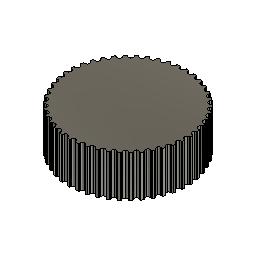
gear_46z (Autodesk Fusion 360 design; units mm, degrees)
Autodesk Fusion 360 part; units mm, degrees
sketch "Sketch1" plane through (0, 0, 0) normal (0, 0, 1) x (1, 0, 0) in component "gt2 pulley"
  circle A0 centre (0, 0) radius 14.6423 construction
  circle A1 centre (0, 0) radius 13.6383 construction
  line L0 (0, 0) -> (0, 14.6423) construction
  line L1 (0, 0) -> (0.9992, 14.6081) construction
  line L2 (0, 0) -> (1.4077, 14.5744) construction
  circle A2 centre (0, 0) radius 14.3883 construction
  arc A3 (0.386, 14.2474) -> (0.4514, 13.9588) centre (1.3833, 14.3216) ccw
  circle A4 centre (0, 0) radius 14.2383 construction
  arc A5 (0.2389, 14.3863) -> (0, 14.3883) centre (0, 0) ccw
  arc A6 (0.386, 14.2474) -> (0.2389, 14.3863) centre (0.2364, 14.2363) ccw
  arc A7 (0.4514, 13.9588) -> (0.9307, 13.6065) centre (0.9686, 14.1602) ccw
  arc A8 (0, 14.3883) -> (-0.2389, 14.3863) centre (0, 0) ccw
  arc A9 (-0.2389, 14.3863) -> (-0.386, 14.2474) centre (-0.2364, 14.2363) ccw
  arc A10 (-0.4514, 13.9588) -> (-0.386, 14.2474) centre (-1.3833, 14.3216) ccw
  arc A11 (-0.9309, 13.6064) -> (-0.4514, 13.9588) centre (-0.9686, 14.1602) ccw
  arc A12 (0.9307, 13.6065) -> (-0.9307, 13.6065) centre (0, 0) ccw
  point P0 (1.3833, 14.3216)
  point P1 (0, 14.3883)
  dimension "d18" = 29.2845
  dimension "d19" = 3.913
  dimension "d22" = 1.004
  dimension "d24" = 0.75
  dimension "d26" = 1
  dimension "d27" = 0.15
  dimension "d28" = 0.15
  dimension "d47" = 0.555
  dimension "d52" = 3.812
  constraint coincident A0.centre A1.centre
  constraint coincident A0 L0.end
  constraint vertical L0
  constraint coincident A0 L1.end
  constraint coincident A0 L2.end
  constraint concentric A1 A2
  constraint coincident A1 A7.end
  constraint coincident L1 A7.end
  constraint coincident A2 P0
  constraint coincident L2 P0
  constraint coincident P0 A3.centre
  constraint coincident A2 P1
  constraint coincident L0 P1
  constraint concentric A2 A4
  constraint coincident P1 A5.end
  constraint coincident A4 A6.centre
  constraint coincident A3.start A6.start
  constraint tangent A3 A6
  constraint tangent A3 A7
  constraint symmetric L0 A7.end A12.end
  constraint symmetric L0 A3.start A9.end
  constraint symmetric L0 A3.end A10.start
  constraint symmetric L0 A3 A10
  constraint symmetric L0 A5.start A8.end
  constraint symmetric L0 P1 A5.end
  constraint symmetric L0 A5 A8
  constraint symmetric L0 A6 A9
  constraint symmetric L0 A7 A11
  constraint coincident A1 A11.start
  constraint tangent A1 A7
  constraint coincident L1 A7.centre
  measures "d18" diameter of A0
  measures "d19" angle of L0 L1
  measures "d22" distance of A0 A1
  measures "d24" distance of A1 A2
  measures "d26" radius of A3
  measures "d27" distance of A2 A4
  measures "d28" radius of A6
  measures "d47" radius of A7
extrude "Extrude1" add sketch "Sketch1" along normal blind 10 makes body 1
pattern_circular "C-Pattern1" count 46 over 360 about axis through (0, 0, 1.75) along (0, 0, 1) of bodies 1 makes body 2 at (-2.572, 13.3935, 6.6667) makes body 3 at (-3.7792, 13.1042, 6.6667) makes body 4 at (-4.7617, 12.78, 3.3333) makes body 5 at (-7.1745, 11.5986, 6.6667) makes body 6 at (-8.0331, 11.0214, 3.3333) makes body 7 at (-9.459, 9.8249, 3.3333) makes body 8 at (-11.544, 7.2621, 6.6667) makes body 9 at (-12.1565, 6.1823, 6.6667) makes body 10 at (-12.5902, 5.243, 3.3333) makes body 11 at (-13.3737, 2.6733, 6.6667) makes body 12 at (-13.5379, 1.6518, 3.3333) makes body 13 at (-13.6367, -0.207, 3.3333) makes body 14 at (-13.1868, -3.48, 6.6667) makes body 15 at (-12.5901, -5.2432, 6.6667) makes body 16 at (-12.4253, -5.6227, 3.3333) makes body 17 at (-11.5439, -7.2623, 3.3333) makes body 18 at (-10.4475, -8.7665, 3.3333) makes body 19 at (-8.033, -11.0215, 6.6667) makes body 20 at (-6.9975, -11.7063, 6.6667) makes body 21 at (-6.09, -12.203, 3.3333) makes body 22 at (-4.3716, -12.9186, 3.3333) makes body 23 at (-2.5718, -13.3936, 3.3333) makes body 24 at (0.1036, -13.6379, 6.6667) makes body 25 at (2.572, -13.3935, 6.6667) makes body 26 at (3.7792, -13.1042, 6.6667) makes body 27 at (4.7617, -12.78, 3.3333) makes body 28 at (7.1745, -11.5986, 6.6667) makes body 29 at (8.0331, -11.0214, 3.3333) makes body 30 at (9.459, -9.8249, 3.3333) makes body 31 at (11.544, -7.2621, 6.6667) makes body 32 at (11.759, -6.9085, 3.3333) makes body 33 at (12.8851, -4.4694, 6.6667) makes body 34 at (13.3737, -2.6733, 6.6667) makes body 35 at (13.5379, -1.6518, 3.3333) makes body 36 at (13.6367, 0.207, 3.3333) makes body 37 at (13.1868, 3.48, 6.6667) makes body 38 at (13.0752, 3.8785, 3.3333) makes body 39 at (12.4253, 5.6227, 3.3333) makes body 40 at (11.5439, 7.2623, 3.3333) makes body 41 at (10.4475, 8.7665, 3.3333) makes body 42 at (8.033, 11.0215, 6.6667) makes body 43 at (7.6949, 11.2601, 3.3333) makes body 44 at (6.09, 12.203, 3.3333) makes body 45 at (4.3716, 12.9186, 3.3333) makes body 46 at (2.5718, 13.3936, 3.3333)
sketch "Sketch2" plane through (0, 0, 10) normal (0, 0, 1) x (-1, 0, 0)
  arc A0 (-10.676, -9.4425) -> (-10.677, -9.6448) centre (-10.5658, -9.5442) ccw
  arc A1 (-10.677, -9.6448) -> (-10.351, -9.994) centre (0, 0) ccw
  arc A2 (-10.351, -9.994) -> (-10.149, -10.0067) centre (-10.243, -9.8898) ccw
  arc A3 (-9.8935, -9.8575) -> (-10.149, -10.0067) centre (-9.5226, -10.7862) ccw
  arc A4 (-9.3088, -9.9673) -> (-9.8935, -9.8575) centre (-9.6876, -10.3729) ccw
  arc A5 (-10.5793, -8.6069) -> (-9.3088, -9.9673) centre (0, 0) ccw
  arc A6 (-10.5097, -9.1977) -> (-10.5793, -8.6069) centre (-11.0099, -8.9572) ccw
  arc A7 (-10.676, -9.4425) -> (-10.5097, -9.1977) centre (-11.4109, -8.7643) ccw
  circle A8 centre (0, 0) radius 13.6383
  constraint concentric A1 A8
extrude "Extrude2" add sketch "Sketch2" against normal blind 10 contours A5 A8 bodies 1 2 3 4 5 6 7 8 9 10 11 12 13 14 15 16 17 18 19 20 21 22 23 24 25 26 27 28 29 30 31 32 33 34 35 36 37 38 39 40 41 42 43 44 45 46
extrude "Extrude4" [suppressed] in component "gt2 pulley"
pattern_circular "C-Pattern7" [suppressed] in component "gt2 pulley"
extrude "Extrude3" [suppressed] in component "gt2 pulley"
pattern_circular "C-Pattern6" [suppressed] in component "gt2 pulley"
extrude "Extrude2'" [suppressed] in component "gt2 pulley"
pattern_circular "C-Pattern5" [suppressed] in component "gt2 pulley"
extrude "Extrude1'" [suppressed] in component "gt2 pulley"
pattern_circular "C-Pattern4" [suppressed] in component "gt2 pulley"
pattern_circular "C-Pattern3" [suppressed] in component "gt2 pulley"
pattern_circular "C-Pattern2" [suppressed] in component "gt2 pulley"
pattern_circular "C-Pattern1'" [suppressed] in component "gt2 pulley"
copy_body "Body->Comp1" [suppressed] in component "Component"
copy_body "Body->Comp2" [suppressed] in component "Component'"
copy_body "Body->Comp3" [suppressed] in component "Component''"
copy_body "Body->Comp4" [suppressed] in component "Component'''"
copy_body "Body->Comp5" [suppressed] in component "Component''''"
copy_body "Body->Comp6" [suppressed] in component "Component'''''"
copy_body "Body->Comp7" [suppressed] in component "Component''''''"
copy_body "Body->Comp8" [suppressed] in component "Component'''''''"
copy_body "Body->Comp9" [suppressed] in component "Component''''''''"
copy_body "Body->Comp10" [suppressed] in component "Component'''''''''"
copy_body "Body->Comp11" [suppressed] in component "Component''''''''''"
copy_body "Body->Comp12" [suppressed] in component "Component'''''''''''"
copy_body "Body->Comp13" [suppressed] in component "Component''''''''''''"
copy_body "Body->Comp14" [suppressed] in component "Component'''''''''''''"
copy_body "Body->Comp15" [suppressed] in component "Component''''''''''''''"
copy_body "Body->Comp16" [suppressed] in component "Component'''''''''''''''"
copy_body "Body->Comp17" [suppressed] in component "Component''''''''''''''''"
copy_body "Body->Comp18" [suppressed] in component "Component'''''''''''''''''"
copy_body "Body->Comp19" [suppressed] in component "Component''''''''''''''''''"
copy_body "Body->Comp20" [suppressed] in component "Component'''''''''''''''''''"
component "gt2 pulley" placed x (1, 0, 0) y (0, 1, 0) z (0, 0, 1) at (0, 0, 0)
equation "NumTeeth = 46" comment "min 20"
equation "ToothPitch = 2 mm"
equation "PullyDia = NumTeeth * ToothPitch / PI"
equation "ToothAng = ( ( 360 / NumTeeth ) * 1 deg )"
equation "TransOffsetAngle = ToothAng * 0.2"
equation "Sholulder_Radius = 0.15 mm"
equation "Root_Radius = 0.555 mm"
equation "TransRadius = 1 mm"
equation "ToolHeight = 0.75 mm"
equation "PLD = 0.254 mm"
equation "d18 = PullyDia"
equation "d19 = ToothAng / 2"
equation "d22 = PLD + ToolHeight"
equation "d24 = ToolHeight"
equation "d26 = TransRadius"
equation "d27 = Sholulder_Radius"
equation "d31 = NumTeeth"
equation "d33 = NumTeeth"
equation "d35 = NumTeeth"
equation "d37 = NumTeeth"
equation "d41 = NumTeeth"
equation "d45 = NumTeeth"
equation "d47 = Root_Radius"
equation "d50 = NumTeeth"
